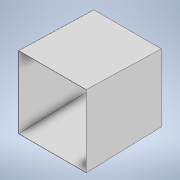
# Autodesk Inventor part: Test Section Ver2
Saved by Autodesk Inventor 2022 (Build 260153000, 153)
## iProperties
Created: 2022-03-08
Part Number: Test Section Ver2
Material: Generic
Document SubType Name: Modeling
Designer: calvi
Density: 1 g/cm^3
Appearance: Default
Author: calvi
Autodesk Inventor part; units mm, degrees
ref_plane "YZ Plane" through (0, 0, 0) normal (1, 0, 0) x (0, 1, 0)
ref_plane "XZ Plane" through (0, 0, 0) normal (0, 1, 0) x (-1, 0, 0)
sketch "Sketch1" plane through (0, 0, 0) normal (0, 0, 1) x (1, 0, 0)
  line L0 (-223.25, 223.25) -> (223.25, 223.25)
  line L1 (-223.25, -223.25) -> (-223.25, 223.25)
  line L2 (223.25, 223.25) -> (223.25, -223.25)
  line L3 (223.25, -223.25) -> (-223.25, -223.25)
  line L4 (224.75, 224.75) -> (-224.75, 224.75)
  line L5 (-224.75, 224.75) -> (-224.75, -224.75)
  line L6 (-224.75, -224.75) -> (224.75, -224.75)
  line L7 (224.75, -224.75) -> (224.75, 224.75)
  point P0 (0, 0)
  point P1 (0, 0)
  dimension "d0" = 1.5
  constraints: 16 end point, 3 other
  measures "d0" distance between parallel lines of L0 L4
ref_plane "Work Plane1" through (0, 0, 500) normal (0, 0, 1) x (1, 0, 0)
sketch "Sketch2" plane through (0, 0, 500) normal (0, 0, 1) x (1, 0, 0)
  line L0 (-223.5, 238.25) -> (223.5, 238.25)
  line L1 (-223.5, -238.25) -> (-223.5, 238.25)
  line L2 (223.5, 238.25) -> (223.5, -238.25)
  line L3 (223.5, -238.25) -> (-223.5, -238.25)
  line L4 (225, 239.75) -> (-225, 239.75)
  line L5 (-225, 239.75) -> (-225, -239.75)
  line L6 (-225, -239.75) -> (225, -239.75)
  line L7 (225, -239.75) -> (225, 239.75)
  point P0 (0, 0)
  point P1 (0, 0)
  dimension "d2" = 1.5
  constraints: 16 end point, 3 other
  measures "d2" distance between parallel lines of L0 L4
loft "Loft1" add profiles "Sketch1", "Sketch2" contours L0 L2 L3 L1 | L7 L6 L5 L4 / L0 L2 L3 L1 | L7 L6 L5 L4
shell "Shell1" thickness 1.5 removed faces 2 at (-75, -79.9167, 500) at (74.9167, -74.9167, 0)
body "Solid1"
